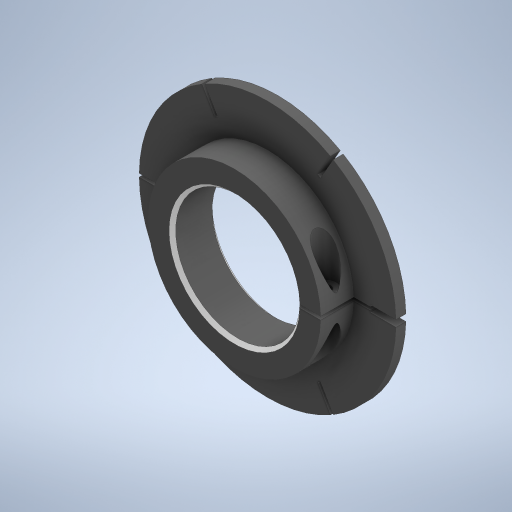
# Autodesk Inventor part: disk_6_slot
Saved by Autodesk Inventor 2023 (Build 270158000, 158)
## iProperties
Created: 2023-10-19
Part Number: disk_6_slot
Material: Generic
Document SubType Name: Modeling
Designer: mark
Density: 1 g/cm^3
Appearance: Default
Author: mark
Autodesk Inventor part; units mm, degrees
ref_plane "YZ Plane" through (0, 0, 0) normal (1, 0, 0) x (0, 1, 0)
ref_plane "XZ Plane" through (0, 0, 0) normal (0, 1, 0) x (-1, 0, 0)
ref_plane "XY Plane" through (0, 0, 0) normal (0, 0, 1) x (1, 0, 0)
sketch "Sketch1" plane through (0, 0, 0) normal (0, 0, 1) x (1, 0, 0)
  circle A0 centre (0, 0) radius 38.75
  line L0 (-0.5, 39) -> (0.5, 39)
  line L1 (0.5, 39) -> (0.5, 31)
  line L2 (0.5, 31) -> (-0.5, 31)
  line L3 (-0.5, 31) -> (-0.5, 39)
  line L4 (-15.933, 26.5968) -> (-19.933, 33.525)
  line L5 (-19.067, 34.025) -> (-15.067, 27.0968)
  line L6 (-15.067, 27.0968) -> (-15.933, 26.5968)
  line L7 (-19.933, 33.525) -> (-19.067, 34.025)
  line L8 (-27.0968, 15.067) -> (-34.025, 19.067)
  line L9 (-33.525, 19.933) -> (-26.5968, 15.933)
  line L10 (-26.5968, 15.933) -> (-27.0968, 15.067)
  line L11 (-34.025, 19.067) -> (-33.525, 19.933)
  line L12 (-31, -0.5) -> (-39, -0.5)
  line L13 (-39, 0.5) -> (-31, 0.5)
  line L14 (-31, 0.5) -> (-31, -0.5)
  line L15 (-39, -0.5) -> (-39, 0.5)
  line L16 (-26.5968, -15.933) -> (-33.525, -19.933)
  line L17 (-34.025, -19.067) -> (-27.0968, -15.067)
  line L18 (-27.0968, -15.067) -> (-26.5968, -15.933)
  line L19 (-33.525, -19.933) -> (-34.025, -19.067)
  line L20 (-15.067, -27.0968) -> (-19.067, -34.025)
  line L21 (-19.933, -33.525) -> (-15.933, -26.5968)
  line L22 (-15.933, -26.5968) -> (-15.067, -27.0968)
  line L23 (-19.067, -34.025) -> (-19.933, -33.525)
  line L24 (0.5, -31) -> (0.5, -39)
  line L25 (-0.5, -39) -> (-0.5, -31)
  line L26 (-0.5, -31) -> (0.5, -31)
  line L27 (0.5, -39) -> (-0.5, -39)
  line L28 (15.933, -26.5968) -> (19.933, -33.525)
  line L29 (19.067, -34.025) -> (15.067, -27.0968)
  line L30 (15.067, -27.0968) -> (15.933, -26.5968)
  line L31 (19.933, -33.525) -> (19.067, -34.025)
  line L32 (27.0968, -15.067) -> (34.025, -19.067)
  line L33 (33.525, -19.933) -> (26.5968, -15.933)
  line L34 (26.5968, -15.933) -> (27.0968, -15.067)
  line L35 (34.025, -19.067) -> (33.525, -19.933)
  line L36 (31, 0.5) -> (39, 0.5)
  line L37 (39, -0.5) -> (31, -0.5)
  line L38 (31, -0.5) -> (31, 0.5)
  line L39 (39, 0.5) -> (39, -0.5)
  line L40 (26.5968, 15.933) -> (33.525, 19.933)
  line L41 (34.025, 19.067) -> (27.0968, 15.067)
  line L42 (27.0968, 15.067) -> (26.5968, 15.933)
  line L43 (33.525, 19.933) -> (34.025, 19.067)
  line L44 (15.067, 27.0968) -> (19.067, 34.025)
  line L45 (19.933, 33.525) -> (15.933, 26.5968)
  line L46 (15.933, 26.5968) -> (15.067, 27.0968)
  line L47 (19.067, 34.025) -> (19.933, 33.525)
  point P0 (0, 31)
  point P1 (-0.5, 38.7468)
  point P2 (0.5, 38.7468)
  point P3 (-15.5, 26.8468)
  point P4 (-26.8468, 15.5)
  point P5 (-31, 0)
  point P6 (-26.8468, -15.5)
  point P7 (-15.5, -26.8468)
  point P8 (0, -31)
  point P9 (15.5, -26.8468)
  point P10 (26.8468, -15.5)
  point P11 (31, 0)
  point P12 (26.8468, 15.5)
  point P13 (15.5, 26.8468)
  point P14 (-18.9404, 33.8057)
  point P15 (-19.8064, 33.3057)
  point P16 (-33.3057, 19.8064)
  point P17 (-33.8057, 18.9404)
  point P18 (-38.7468, 0.5)
  point P19 (-38.7468, -0.5)
  point P20 (-33.8057, -18.9404)
  point P21 (-33.3057, -19.8064)
  point P22 (-19.8064, -33.3057)
  point P23 (-18.9404, -33.8057)
  point P24 (-0.5, -38.7468)
  point P25 (0.5, -38.7468)
  point P26 (18.9404, -33.8057)
  point P27 (19.8064, -33.3057)
  point P28 (33.3057, -19.8064)
  point P29 (33.8057, -18.9404)
  point P30 (38.7468, -0.5)
  point P31 (38.7468, 0.5)
  point P32 (33.8057, 18.9404)
  point P33 (33.3057, 19.8064)
  point P34 (19.8064, 33.3057)
  point P35 (18.9404, 33.8057)
  dimension "d0" = 77.5
  dimension "d3" = 0.5
  dimension "d4" = 31
  dimension "d9" = 360
  constraints: 96 end point, 2 parallel, 1 coincident, 1 horizontal, 1 midpoint, 1 perpendicular, 111 other
  measures "d3" distance from line of point (0, 0) L1
  measures "d4" distance of point (0, 0) point (0, 31)
extrude "Extrusion1" add sketch "Sketch1" along normal blind 3 contours L36 L38 L37 A0 L32 L34 L33 L28 L30 L29 L24 L26 L25 L20 L22 L21 L16 L18 L17 L12 L14 L13 L8 L10 L9 L4 L6 L5 L3 L2 L1 L44 L46 L45 L40 L42 L41 | L41 L42 L40 A0 | A0 L40 L43 L41 | L32 L35 L33 A0 | A0 L33 L34 L32 | L1 L2 L3 A0 | A0 L3 L0 L1 | L24 L27 L25 A0 | A0 L25 L26 L24 | L9 L10 L8 A0 | A0 L8 L11 L9 | L16 L19 L17 A0 | A0 L17 L18 L16
sketch "Sketch2" plane through (0, 0, 3) normal (0, 0, 1) x (1, 0, 0)
  circle A0 centre (0, 0) radius 18.75
  circle A1 centre (0, 0) radius 26
  dimension "d11" = 37.5
  dimension "d12" = 52
  constraints: 2 centre point, 2 coincident
  measures "d11" diameter of A0
  measures "d12" diameter of A1
extrude "Extrusion2" add sketch "Sketch2" along normal blind 10
sketch "Sketch3" plane through (0, 0, 3) normal (0, 0, 1) x (1, 0, 0)
  circle A0 centre (0, 0) radius 18.75
  constraints: 1 centre point, 1 coincident
extrude "Extrusion3" cut sketch "Sketch3" against normal blind 10
sketch "Sketch4" plane through (0, 0, 13) normal (0, 0, 1) x (1, 0, 0)
  arc A0 (33.8057, -18.9404) -> (38.7468, -0.5) centre (0, 0) ccw projected
  line L0 (38.7468, -0.5) -> (17.4484, -0.5)
  line L1 (17.4484, -0.5) -> (17.4484, 0.5)
  line L2 (17.4484, 0.5) -> (38.7468, 0.5)
  line L3 (38.7468, 0.5) -> (38.7468, -0.5)
  line L4 (31, 1) -> (40.0251, 1)
  line L5 (40.0251, 1) -> (40.0251, -1)
  line L6 (40.0251, -1) -> (31, -1)
  line L7 (31, -1) -> (31, 1)
  point P0 (31, -0.5)
  point P1 (31, 0.5)
  dimension "d19" = 2
  dimension "d20" = 0.5
  constraints: 16 end point, 4 parallel, 2 horizontal, 2 perpendicular
  measures "d19" distance of L4.end L5.end
  measures "d20" distance between parallel lines of L2 L4
extrude "Extrusion4" cut sketch "Sketch4" against normal through all
sketch "Sketch5" plane through (18.7433, 0.5, 13) normal (0, -1, 0) x (1, 0, 0)
  circle A0 centre (3.7, -5) radius 1.6
  line L0 (14.5624, -10) -> (1.0631, -10) projected
  line L1 (-37.4933, 0) -> (0, 0) projected
  line L2 (0, 0) -> (0, -10)
  point P0 (-18.7433, -13)
  point P1 (0, -5)
  dimension "d21" = 3.2
  dimension "d22" = 5
  dimension "d23" = 3.7
  constraints: 2 end point, 1 centre point, 1 midpoint, 1 vertical
  measures "d21" diameter of A0
  measures "d22" distance from line of L0 A0.centre
  measures "d23" distance of point (0, -5) A0.centre
extrude "Extrusion5" cut sketch "Sketch5" against normal blind 23.5
ref_plane "Work Plane1" through (18.7433, 3.5, 13) normal (0, -1, 0) x (1, 0, 0)
sketch "Sketch6" plane through (18.7433, 3.5, 13) normal (0, -1, 0) x (1, 0, 0)
  circle A0 centre (3.7, -5) radius 1.6 projected
  circle A1 centre (3.7, -5) radius 3.25
  point P0 (-18.7433, -13)
  dimension "d27" = 6.5
  constraints: 1 centre point, 1 coincident
  measures "d27" diameter of A1
extrude "Extrusion6" cut sketch "Sketch6" against normal blind 23.5
mirror "Mirror1" about plane through (0, 0, 0) normal (0, 1, 0) of "Extrusion6", "Extrusion5"
chamfer "Chamfer1" distance 1 angle 45 2 edges at (-18.75, 0, 13) (-18.75, 0, 0)
sketch "Sketch7" plane through (0, 0, 3) normal (0, 0, 1) x (1, 0, 0)
  circle A0 centre (0, 0) radius 38.75
  arc A1 (18.9404, 33.8057) -> (0.5, 38.7468) centre (0, 0) ccw projected
  circle A2 centre (0, 0) radius 41.405
  constraints: 2 centre point, 2 coincident
extrude "Extrusion7" cut sketch "Sketch7" against normal blind 3
body "Solid1"
